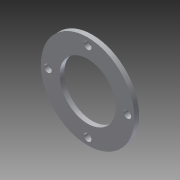
# Autodesk Inventor part: P80 Spacer
Saved by Autodesk Inventor 2013 (Build 170138000, 138)
## iProperties
Created: 2013-02-10
Part Number: P80 Spacer
Material: Aluminum 6061
Document SubType Name: Modeling
Designer: Moses
Mass: 16.7418 g
Surface Area: 51.0761 cm^2
Volume: 6.17778 cm^3
Density: 2.71 g/cm^3
Author: Moses
Autodesk Inventor part; units mm, degrees
ref_plane "YZ Plane" through (0, 0, 0) normal (1, 0, 0) x (0, 1, 0)
ref_plane "XZ Plane" through (0, 0, 0) normal (0, 1, 0) x (-1, 0, 0)
ref_plane "XY Plane" through (0, 0, 0) normal (0, 0, 1) x (1, 0, 0)
sketch "Sketch1" plane through (0, 0, 0) normal (0, 0, 1) x (1, 0, 0)
  circle A0 centre (0, 0) radius 19.05
  circle A1 centre (0, 0) radius 31.75
  circle A2 centre (-27.0002, 0) radius 2.54
  line L0 (-27.0002, 0) -> (0, 0) construction
  circle A3 centre (0, -27.0002) radius 2.54
  circle A4 centre (27.0002, 0) radius 2.54
  circle A5 centre (0, 27.0002) radius 2.54
  dimension "d0" = 63.5
  dimension "d2" = 38.1
  dimension "d3" = 27.0002
  dimension "d4" = 5.08
  dimension "d7" = 360
  constraints: 6 centre point, 2 coincident, 2 end point, 1 horizontal, 9 other
  measures "d0" diameter of A1
  measures "d2" diameter of A0
  measures "d3" distance of L0.start L0.end
  measures "d4" diameter of A2
extrude "Extrusion1" add sketch "Sketch1" along normal blind 3.175
body "Solid1"
